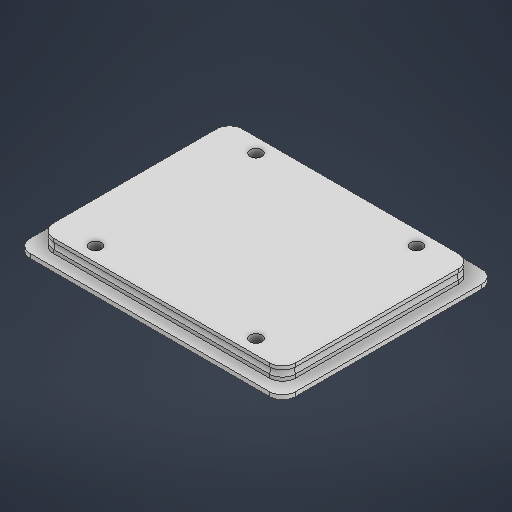
# Autodesk Inventor part: Lid
Saved by Autodesk Inventor 2026 (Build 300175000, 175)
## iProperties
Created: 2025-05-11
Part Number: Lid
Material: Generic
Document SubType Name: Modeling
Designer: Riley
Density: 1 g/cm^3
Appearance: Default
Author: Riley
Autodesk Inventor part; units mm, degrees
ref_plane "YZ Plane" through (0, 0, 0) normal (1, 0, 0) x (0, 1, 0)
ref_plane "XZ Plane" through (0, 0, 0) normal (0, 1, 0) x (-1, 0, 0)
ref_plane "XY Plane" through (0, 0, 0) normal (0, 0, 1) x (1, 0, 0)
sketch "Sketch1" plane through (0, 0, 0) normal (0, 1, 0) x (-1, 0, 0)
  line L0 (0, 0) -> (100, 0)
  line L1 (100, 0) -> (100, -80)
  line L2 (100, -80) -> (0, -80)
  line L3 (0, -80) -> (0, 0)
  dimension "d0" = 100
  dimension "d1" = 80
  constraints: 8 end point, 2 parallel, 1 horizontal, 1 perpendicular
  measures "d0" distance of L1.end L2.end
  measures "d1" distance of L0.end L1.end
extrude "LidBase" add sketch "Sketch1" along normal blind 1.6
fillet "Fillet1" radius 5 4 edges at (-100, 0.8, 0) (0, 0.8, 0) (0, 0.8, -80) (-100, 0.8, -80)
sketch "Sketch3" plane through (0, 1.6, 0) normal (0, 1, 0) x (1, 0, 0)
  line L0 (-5, 80) -> (-95, 80) projected
  arc A0 (-95, 80) -> (-100, 75) centre (-95, 75) ccw projected
  line L1 (-100, 75) -> (-100, 5) projected
  arc A1 (-100, 5) -> (-95, 0) centre (-95, 5) ccw projected
  line L2 (-95, 0) -> (-5, 0) projected
  arc A2 (-5, 0) -> (0, 5) centre (-5, 5) ccw projected
  line L3 (0, 5) -> (0, 75) projected
  arc A3 (0, 75) -> (-5, 80) centre (-5, 75) ccw projected
  line L4 (-5, 80) -> (-95, 80) projected
  line L5 (-95.6, 75.6) -> (-4.4, 75.6)
  line L6 (-4.4, 75.6) -> (-4.4, 4.4)
  line L7 (-4.4, 4.4) -> (-95.6, 4.4)
  line L8 (-95.6, 4.4) -> (-95.6, 75.6)
  point P0 (0, 0)
  dimension "d5" = 4.4
  dimension "d6" = 4.4
  dimension "d7" = 4.4
  dimension "d8" = 4.4
  constraints: 8 end point, 2 parallel, 1 horizontal, 1 perpendicular
  measures "d5" distance between parallel lines of L3 L6
  measures "d6" distance between parallel lines of L1 L8
  measures "d7" distance between parallel lines of L0 L5
  measures "d8" distance between parallel lines of L2 L7
extrude "Gasket Seal" add sketch "Sketch3" along normal blind 5 contours L5 L6 L7 L8
fillet "Fillet2" radius 5 4 edges at (-4.4, 4.1, -4.4) (-4.4, 4.1, -75.6) (-95.6, 4.1, -75.6) (-95.6, 4.1, -4.4)
ref_plane "Work Plane4" through (-54.4, 1.6, -9.4) normal (1, 0, 0) x (0, 0, -1)
sketch "Sketch7" plane through (-54.4, 1.6, -9.4) normal (1, 0, 0) x (0, 0, -1)
  line L0 (70.6, -1.6) -> (-9.4, -1.6) projected
  line L1 (-9.4, -1.6) -> (-9.4, 0) projected
  line L2 (-9.4, 0) -> (-5, 0) projected
  line L3 (-5, 0) -> (-5, 5) projected
  line L4 (-5, 5) -> (66.2, 5) projected
  line L5 (66.2, 5) -> (66.2, 0) projected
  line L6 (66.2, 0) -> (70.6, 0) projected
  line L7 (70.6, 0) -> (70.6, -1.6) projected
  circle A0 centre (-6.1, 2.5) radius 1.6
  point P0 (-9.4, -1.6)
  dimension "d24" = 3.2
  dimension "d25" = 2.5
  dimension "d26" = 1.1
  constraints: 1 centre point
  measures "d24" diameter of A0
  measures "d25" distance from line of A0.centre L4
  measures "d26" distance from line of L3 A0.centre
sketch3d "3D Sketch3"
  line L0 (-90.6, 1.6, -4.4) -> (-9.4, 1.6, -4.4)
  arc A0 (-9.4, 1.6, -4.4) -> (-4.4, 1.6, -9.4) centre (-9.4, 1.6, -9.4) ccw
  line L1 (-4.4, 1.6, -9.4) -> (-4.4, 1.6, -70.6)
  arc A1 (-4.4, 1.6, -70.6) -> (-9.4, 1.6, -75.6) centre (-9.4, 1.6, -70.6) ccw
  line L2 (-9.4, 1.6, -75.6) -> (-90.6, 1.6, -75.6)
  arc A2 (-90.6, 1.6, -75.6) -> (-95.6, 1.6, -70.6) centre (-90.6, 1.6, -70.6) ccw
  line L3 (-95.6, 1.6, -70.6) -> (-95.6, 1.6, -9.4)
  arc A3 (-95.6, 1.6, -9.4) -> (-90.6, 1.6, -4.4) centre (-90.6, 1.6, -9.4) ccw
sweep "Oring Channel" cut profiles "Sketch7" path "3D Sketch3" contours A0 L3 | L3 A0
sketch "Sketch8" plane through (0, 0, 0) normal (0, 1, 0) x (1, 0, 0)
  line L0 (-100, 75) -> (-100, 5) projected
  line L1 (-95, 0) -> (-5, 0) projected
  line L2 (-9.4, 75.6) -> (-90.6, 75.6) projected
  line L3 (-5, 80) -> (-95, 80) projected
  line L4 (0, 5) -> (0, 75) projected
  point P0 (0, 0)
  point P1 (-80.2, 9.8)
  point P2 (-19.8, 9.8)
  point P3 (-19.8, 70.2)
  point P4 (-80.2, 70.2)
  dimension "d29" = 19.8
  dimension "d30" = 9.8
  dimension "d32" = 9.8
  dimension "d33" = 19.8
  dimension "d34" = 19.8
  dimension "d35" = 9.8
  dimension "d36" = 19.8
  dimension "d37" = 9.8
  measures "d29" distance from line of L0 point (-80.2, 9.8)
  measures "d30" distance from line of L1 point (-80.2, 9.8)
  measures "d32" distance from line of L3 point (-80.2, 70.2)
  measures "d33" distance from line of L0 point (-80.2, 70.2)
  measures "d34" distance from line of L4 point (-19.8, 9.8)
  measures "d35" distance from line of L1 point (-19.8, 9.8)
  measures "d36" distance from line of L4 point (-19.8, 70.2)
  measures "d37" distance from line of L3 point (-19.8, 70.2)
hole "Hole1" at (-80.2, 0, -9.8) at (-19.8, 0, -9.8) at (-19.8, 0, -70.2) at (-80.2, 0, -70.2) direction (0, 1, 0) diameter 4.4 end through all counterbore diameter 8.2 counterbore depth 3.2
equation "\"d6\" = d5"
equation "\"d7\" = d5"
equation "\"d8\" = d5"
equation "\"d32\" = d30"
equation "\"d33\" = d29"
equation "\"d34\" = d29"
equation "\"d35\" = d30"
equation "\"d36\" = d34"
equation "\"d37\" = d30"
body "Solid1"
